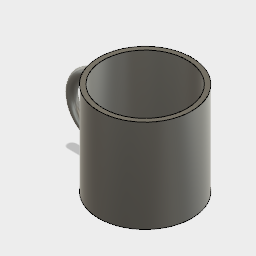
水杯 (Autodesk Fusion 360 design; units mm, degrees)
Autodesk Fusion 360 part; units mm, degrees
cylinder "圆柱体基本要素1" add diameter 20 height 20 placed x (1, 0, 0) y (0, 0, -1) z (0, 1, 0) at (65, 0, 70) makes body 1
cylinder "圆柱体基本要素2" add diameter 18 height 20 placed x (1, 0, 0) y (0, 0, -1) z (0, 1, 0) at (101.1106, 0, 38.307) separate body makes body 2
torus "圆环体基本要素1" add centre line diameter 12 section diameter 2 placed x (1, 0, 0) y (0, 0, -1) z (0, 1, 0) at (40, 0, 15) separate body makes body 3
delete_face "删除面1" 1 faces at (46.3948, 0.342, 12.3044) on bodies 3
torus "圆环体基本要素2" add centre line diameter 12 section diameter 2 placed x (1, 0, 0) y (0, 1, 0) z (0, 0, 1) at (64.1807, 12.2148, 0) separate body makes body 4
move_body "MoveFace1" bodies 4 to x (1, 0, 0) y (0, 1, 0) z (0, 0, 1) at (18.8993, 15.6267, 7.0719) on bodies 4
move_body "MoveFace2" bodies 4 to x (1, 0, 0) y (0, 1, 0) z (0, 0, 1) at (3.7259, 7.6315, 15.5905) on bodies 4
move_body "MoveFace3" bodies 4 to x (1, 0, 0) y (0, 1, 0) z (0, 0, 1) at (5.0421, 0, 15.7079) on bodies 4
move_body "MoveFace4" bodies 4 to x (1, 0, 0) y (0, 1, 0) z (0, 0, 1) at (-37.2336, -25.4042, 0) on bodies 4
move_body "MoveFace5" bodies 4 to x (1, 0, 0) y (0, 1, 0) z (0, 0, 1) at (0, 0, 31) on bodies 4
combine "合并1" operation add target body 1 tool bodies 4
move_body "移动1" bodies 2 to x (1, 0, 0) y (0, 1, 0) z (0, 0, 1) at (-36.0582, 27.2084, 0)
move_body "移动2" bodies 2 to x (1, 0, 0) y (0, 1, 0) z (0, 0, 1) at (0, 0, 32)
move_body "对齐1" bodies 2 to x (1, 0, 0) y (0, 1, 0) z (0, 0, 1) at (-0.0524, -27.2084, -0.307)
move_face "偏移面1" offset -2 1 faces at (64.3918, 0, 71.9478) on bodies 2
combine "合并2" operation cut target body 1 tool bodies 2
